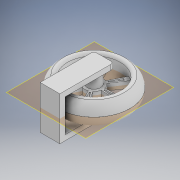
# Autodesk Inventor part: PrednjiKotač_v.1.0
Saved by Autodesk Inventor 2020 (Build 240168000, 168)
## iProperties
Created: 2020-07-15
Part Number: PrednjiKotač_v.1.0
Material: Generic
Document SubType Name: Modeling
Designer: Sičaja
Density: 1 g/cm^3
Appearance: Default
Author: Sičaja
Autodesk Inventor part; units mm, degrees
ref_plane "YZ Plane" through (0, 0, 0) normal (1, 0, 0) x (0, 1, 0)
ref_plane "XZ Plane" through (0, 0, 0) normal (0, 1, 0) x (-1, 0, 0)
ref_plane "XY Plane" through (0, 0, 0) normal (0, 0, 1) x (1, 0, 0)
sketch "Sketch1" plane through (0, 0, 0) normal (0, 1, 0) x (-1, 0, 0)
  circle A0 centre (0, 0) radius 13.75
  circle A1 centre (0, 0) radius 1
  circle A2 centre (0, 0) radius 10.0126
  line L0 (9.6185, 1) -> (0.866, 0.5)
  line L1 (9.6185, -1) -> (0.866, -0.5)
  line L2 (9.6185, -1) -> (9.9605, -1.0195)
  line L3 (9.6185, 1) -> (9.9605, 1.0195)
  line L4 (3.9765, -0.2067) -> (3.953, 0.2053)
  line L5 (8.3776, -0.4581) -> (3.9765, -0.2067)
  line L6 (8.3776, 0.4581) -> (3.953, 0.2053)
  line L7 (8.3776, 0) -> (8.3776, -0.4581)
  line L8 (8.8989, -0.9589) -> (8.8989, -1)
  line L9 (8.8989, 1) -> (8.8989, 0.9589)
  line L10 (8.3776, 0.4581) -> (8.3776, 0)
  line L11 (3.9432, 8.8299) -> (4.0973, 9.1359)
  line L12 (5.6753, 7.8299) -> (5.8632, 8.1163)
  line L13 (5.6753, 7.8299) -> (0.866, 0.5)
  line L14 (3.9432, 8.8299) -> (0, 1)
  line L15 (4.1888, 7.2552) -> (4.5855, 7.0261)
  line L16 (3.7921, 7.4842) -> (4.1888, 7.2552)
  line L17 (3.7921, 7.4842) -> (1.7987, 3.5261)
  line L18 (4.5855, 7.0261) -> (2.1672, 3.3405)
  line L19 (2.1672, 3.3405) -> (1.7987, 3.5261)
  line L20 (-5.6753, 7.8299) -> (-5.8632, 8.1163)
  line L21 (-3.9432, 8.8299) -> (-4.0973, 9.1359)
  line L22 (-3.9432, 8.8299) -> (0, 1)
  line L23 (-5.6753, 7.8299) -> (-0.866, 0.5)
  line L24 (-4.1888, 7.2552) -> (-3.7921, 7.4842)
  line L25 (-4.5855, 7.0261) -> (-4.1888, 7.2552)
  line L26 (-4.5855, 7.0261) -> (-2.1543, 3.3207)
  line L27 (-3.7921, 7.4842) -> (-1.8093, 3.5471)
  line L28 (-1.8093, 3.5471) -> (-2.1543, 3.3207)
  line L29 (-9.6185, -1) -> (-9.9605, -1.0195)
  line L30 (-9.6185, 1) -> (-9.9605, 1.0195)
  line L31 (-9.6185, 1) -> (-0.866, 0.5)
  line L32 (-9.6185, -1) -> (-0.866, -0.5)
  line L33 (-8.3776, 0) -> (-8.3776, 0.4581)
  line L34 (-8.3776, -0.4581) -> (-8.3776, 0)
  line L35 (-8.3776, -0.4581) -> (-3.953, -0.2053)
  line L36 (-8.3776, 0.4581) -> (-3.9765, 0.2067)
  line L37 (-3.9765, 0.2067) -> (-3.953, -0.2053)
  line L38 (-3.9432, -8.8299) -> (-4.0973, -9.1359)
  line L39 (-5.6753, -7.8299) -> (-5.8632, -8.1163)
  line L40 (-5.6753, -7.8299) -> (-0.866, -0.5)
  line L41 (-3.9432, -8.8299) -> (0, -1)
  line L42 (-4.1888, -7.2552) -> (-4.5855, -7.0261)
  line L43 (-3.7921, -7.4842) -> (-4.1888, -7.2552)
  line L44 (-3.7921, -7.4842) -> (-1.7987, -3.5261)
  line L45 (-4.5855, -7.0261) -> (-2.1672, -3.3405)
  line L46 (-2.1672, -3.3405) -> (-1.7987, -3.5261)
  line L47 (5.6753, -7.8299) -> (5.8632, -8.1163)
  line L48 (3.9432, -8.8299) -> (4.0973, -9.1359)
  line L49 (3.9432, -8.8299) -> (0, -1)
  line L50 (5.6753, -7.8299) -> (0.866, -0.5)
  line L51 (4.1888, -7.2552) -> (3.7921, -7.4842)
  line L52 (4.5855, -7.0261) -> (4.1888, -7.2552)
  line L53 (4.5855, -7.0261) -> (2.1543, -3.3207)
  line L54 (3.7921, -7.4842) -> (1.8093, -3.5471)
  line L55 (1.8093, -3.5471) -> (2.1543, -3.3207)
  circle A3 centre (0, 0) radius 2.25
  circle A4 centre (0, 0) radius 2.25
  point P0 (5.2799, 7.2273)
  point P1 (3.619, 8.1862)
  point P2 (-3.619, 8.1862)
  point P3 (-5.2799, 7.2273)
  point P4 (-8.8989, 0.9589)
  point P5 (-8.8989, -0.9589)
  point P6 (-5.2799, -7.2273)
  point P7 (-3.619, -8.1862)
  point P8 (3.619, -8.1862)
  point P9 (5.2799, -7.2273)
  dimension "d0" = 27.5
  dimension "d1" = 2
  dimension "d12" = 360
  dimension "d14" = 4.5
  constraints: 112 end point, 24 point on line, 5 centre point, 5 coincident, 4 point on circle, 2 parallel, 1 concentric, 1 perpendicular, 133 other
  measures "d0" diameter of A0
  measures "d1" diameter of A1
  measures "d14" diameter of A3
sketch "Sketch4" plane through (0, 0, 0) normal (0, 1, 0) x (-1, 0, 0)
  circle A0 centre (0, 0) radius 2.5
  line L0 (9.6185, 1) -> (0.866, 0.5) projected
  line L1 (8.3776, 0.4581) -> (3.953, 0.2053) projected
  line L2 (8.3776, 0.4581) -> (8.3776, 0) projected
  line L3 (8.3776, 0) -> (8.3776, -0.4581) projected
  line L4 (9.6185, -1) -> (0.866, -0.5) projected
  line L5 (9.6185, -1) -> (9.9605, -1.0195) projected
  line L6 (9.6185, 1) -> (9.9605, 1.0195) projected
  line L7 (3.9765, -0.2067) -> (3.953, 0.2053) projected
  line L8 (8.3776, -0.4581) -> (3.9765, -0.2067) projected
  line L9 (2.9356, -0.6182) -> (9.9605, -1.0195)
  line L10 (2.9356, 0.6182) -> (9.9605, 1.0195)
  circle A1 centre (0, 0) radius 10.0126 projected
  circle A2 centre (0, 0) radius 10.0126
  line L11 (3.953, 0.2053) -> (3.9765, -0.2067)
  line L12 (8.3776, -0.4581) -> (8.3776, 0.4581)
  line L13 (8.3776, 0.4581) -> (3.953, 0.2053)
  line L14 (3.9765, -0.2067) -> (8.3776, -0.4581)
  line L15 (0.9324, 2.8514) -> (4.0973, 9.1359)
  line L16 (3.7921, 7.4842) -> (1.7987, 3.5261)
  line L17 (2.1672, 3.3405) -> (4.5855, 7.0261)
  line L18 (2.0032, 2.2332) -> (5.8632, 8.1163)
  line L19 (4.5855, 7.0261) -> (3.7921, 7.4842)
  line L20 (1.7987, 3.5261) -> (2.1672, 3.3405)
  line L21 (-2.0032, 2.2332) -> (-5.8632, 8.1163)
  line L22 (-4.5855, 7.0261) -> (-2.1543, 3.3207)
  line L23 (-1.8093, 3.5471) -> (-3.7921, 7.4842)
  line L24 (-0.9324, 2.8514) -> (-4.0973, 9.1359)
  line L25 (-3.7921, 7.4842) -> (-4.5855, 7.0261)
  line L26 (-2.1543, 3.3207) -> (-1.8093, 3.5471)
  line L27 (-2.9356, -0.6182) -> (-9.9605, -1.0195)
  line L28 (-8.3776, -0.4581) -> (-3.953, -0.2053)
  line L29 (-3.9765, 0.2067) -> (-8.3776, 0.4581)
  line L30 (-2.9356, 0.6182) -> (-9.9605, 1.0195)
  line L31 (-8.3776, 0.4581) -> (-8.3776, -0.4581)
  line L32 (-3.953, -0.2053) -> (-3.9765, 0.2067)
  line L33 (-0.9324, -2.8514) -> (-4.0973, -9.1359)
  line L34 (-3.7921, -7.4842) -> (-1.7987, -3.5261)
  line L35 (-2.1672, -3.3405) -> (-4.5855, -7.0261)
  line L36 (-2.0032, -2.2332) -> (-5.8632, -8.1163)
  line L37 (-4.5855, -7.0261) -> (-3.7921, -7.4842)
  line L38 (-1.7987, -3.5261) -> (-2.1672, -3.3405)
  line L39 (2.0032, -2.2332) -> (5.8632, -8.1163)
  line L40 (4.5855, -7.0261) -> (2.1543, -3.3207)
  line L41 (1.8093, -3.5471) -> (3.7921, -7.4842)
  line L42 (0.9324, -2.8514) -> (4.0973, -9.1359)
  line L43 (3.7921, -7.4842) -> (4.5855, -7.0261)
  line L44 (2.1543, -3.3207) -> (1.8093, -3.5471)
  arc A3 (2.9356, 0.6182) -> (2.0032, 2.2332) centre (0, 0) ccw
  arc A4 (0.9324, 2.8514) -> (-0.9324, 2.8514) centre (0, 0) ccw
  arc A5 (-2.0032, 2.2332) -> (-2.9356, 0.6182) centre (0, 0) ccw
  arc A6 (-2.9356, -0.6182) -> (-2.0032, -2.2332) centre (0, 0) ccw
  arc A7 (-0.9324, -2.8514) -> (0.9324, -2.8514) centre (0, 0) ccw
  arc A8 (2.0032, -2.2332) -> (2.9356, -0.6182) centre (0, 0) ccw
  circle A9 centre (0, 0) radius 3.5
  point P0 (-9.9605, 1.0195)
  point P1 (-9.9605, -1.0195)
  point P2 (-5.8632, -8.1163)
  point P3 (-4.0973, -9.1359)
  point P4 (3.4397, 0.647)
  point P5 (2.2802, 2.6553)
  point P6 (1.1595, 3.3024)
  point P7 (-1.1595, 3.3024)
  point P8 (2.2802, -2.6553)
  point P9 (3.4397, -0.647)
  point P10 (-1.1595, -3.3024)
  point P11 (1.1595, -3.3024)
  point P12 (-3.4397, -0.647)
  point P13 (-2.2802, -2.6553)
  point P14 (-2.2802, 2.6553)
  point P15 (-3.4397, 0.647)
  dimension "d17" = 5
  dimension "d21" = 360
  dimension "d28" = 7
  constraints: 72 end point, 12 point on circle, 9 centre point, 4 coincident, 4 collinear, 2 point on line, 1 concentric, 1 perpendicular, 85 other
  measures "d17" diameter of A0
  measures "d28" diameter of A9
extrude "Extrusion1" add sketch "Sketch4" along normal mid plane 2.5 contours A0 L0 A9 L4 | A0 L4 A8 L39 A9 L42 A7 L33 L36 A6 L27 L30 A5 L21 L24 A4 L15 L18 A3 L0 | A3 L18 A9 L0 | L4 A9 L39 A8 | L0 L6 A1 L5 L4 A9 | A9 L15 A1 L18 | L39 A1 L42 A9 | L15 A4 L24 A9 | A9 L33 A7 L42 | A9 L21 A1 L24 | L33 A1 L36 A9 | L21 A5 L30 A9 | A9 L27 A6 L36 | A9 L27 A1 L30
extrude "Extrusion2" add sketch "Sketch1" along normal mid plane 10 contours A0
fillet "Fillet1" radius 5.2 2 edges at (13.75, 5, 0) (13.75, -5, 0)
sketch "Sketch5" plane through (0, 1.25, 0) normal (0, 1, 0) x (1, 0, 0)
  circle A0 centre (0, 0) radius 2.5
  circle A1 centre (0, 0) radius 3.5
  circle A2 centre (0, 0) radius 2.5 projected
  circle A3 centre (0, 0) radius 1.25
  dimension "d29" = 2.5
  constraints: 3 centre point, 3 coincident
  measures "d29" diameter of A3
fillet "Fillet2" radius 1 1 edges at (10.0126, 5, 0)
extrude "Extrusion3" add sketch "Sketch5" along normal blind 5 contours A0
sketch "Sketch6" plane through (0, 6.25, 0) normal (0, 1, 0) x (1, 0, 0)
  line L0 (-3.75, 3.75) -> (3.75, 3.75)
  line L1 (3.75, 3.75) -> (3.75, -3.75)
  line L2 (-3.75, -3.75) -> (-3.75, 3.75)
  line L3 (-3.75, 3.75) -> (3.75, -3.75) construction
  line L4 (3.75, 3.75) -> (-3.75, -3.75) construction
  line L5 (-3.75, -3.75) -> (-3.75, -14.75)
  line L6 (-3.75, -14.75) -> (3.75, -14.75)
  line L7 (3.75, -14.75) -> (3.75, -3.75)
  line L8 (-3.75, -14.75) -> (-3.75, -16.75)
  line L9 (-3.75, -16.75) -> (3.75, -16.75)
  line L10 (3.75, -16.75) -> (3.75, -14.75)
  point P0 (0, 0)
  dimension "d33" = 7.5
  dimension "d34" = 7.5
  dimension "d35" = 11
  dimension "d36" = 7.5
  dimension "d37" = 2
  constraints: 22 end point, 3 perpendicular, 2 horizontal, 2 midpoint, 1 parallel, 1 point on line, 1 vertical
  measures "d33" distance of L1.end L2.start
  measures "d34" distance of L0.end L1.end
  measures "d35" distance of L2.start L5.end
  measures "d36" distance of L5.end L6.end
  measures "d37" distance of L5.end L8.end
extrude "Extrusion4" add sketch "Sketch6" along normal blind 2
fillet "Fillet3" radius 1 2 edges at (-3.75, 7.25, -3.75) (3.75, 7.25, -3.75)
sketch "Sketch7" plane through (0, 6.25, 0) normal (0, -1, 0) x (1, 0, 0)
  line L0 (-3.75, 16.75) -> (3.75, 16.75) projected
  line L1 (-3.75, 16.75) -> (-3.75, 14.75)
  line L2 (-3.75, -2.75) -> (-3.75, 16.75) projected
  line L3 (-3.75, 14.75) -> (3.75, 14.75)
  line L4 (3.75, 16.75) -> (3.75, -2.75) projected
  line L5 (3.75, 16.75) -> (-3.75, 16.75)
  point P0 (0, 0)
  dimension "d41" = 2
  constraints: 6 end point, 2 point on line, 1 parallel, 1 perpendicular
  measures "d41" distance of L0.start L1.end
extrude "Extrusion5" add sketch "Sketch7" along normal blind 6.26
ref_plane "Work Plane1" through (0, 0, 0) normal (0, 1, 0) x (1, 0, 0)
mirror "Mirror1" about plane through (0, 0, 0) normal (0, 1, 0) of "Extrusion4", "Extrusion5"
body "Solid1"
